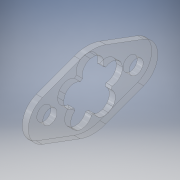
# Autodesk Inventor part: Ball Bearing Center
Saved by Autodesk Inventor 2017 (Build 210142000, 142)
## iProperties
Created: 2018-05-11
Part Number: Ball Bearing Center
Material: Polycarbonate, Clear
Document SubType Name: Modeling
Designer: Steven
Density: 1.2 g/cm^3
Appearance: Polycarbonate - Clear
Author: Steven
Autodesk Inventor part; units mm, degrees
ref_plane "YZ Plane" through (0, 0, 0) normal (1, 0, 0) x (0, 1, 0)
ref_plane "XZ Plane" through (0, 0, 0) normal (0, 1, 0) x (-1, 0, 0)
ref_plane "XY Plane" through (0, 0, 0) normal (0, 0, 1) x (1, 0, 0)
sketch "Sketch1" plane through (0, 0, 0) normal (1, 0, 0) x (0, 1, 0)
  circle A0 centre (0, 0) radius 8.89
  circle A1 centre (0, 0) radius 10.795 construction
  line L0 (0, 0) -> (0, 12.7)
  line L1 (0, 0) -> (0, -12.7)
  circle A2 centre (0, -12.7) radius 2.0955
  circle A3 centre (0, 12.7) radius 2.0955
  circle A4 centre (0, 12.7) radius 6.35 construction
  circle A5 centre (0, -12.7) radius 6.35 construction
  line L2 (5.9484, 14.9225) -> (10.1122, 3.7782)
  line L3 (10.1122, -3.7783) -> (5.9484, -14.9225)
  line L4 (-5.9484, -14.9225) -> (-10.1122, -3.7782)
  line L5 (-5.9484, 14.9225) -> (-10.1122, 3.7782)
  arc A6 (5.9484, 14.9225) -> (-5.9484, 14.9225) centre (0, 12.7) ccw
  arc A7 (10.1122, -3.7783) -> (10.1122, 3.7782) centre (0, 0) ccw
  arc A8 (-5.9484, -14.9225) -> (5.9484, -14.9225) centre (0, -12.7) ccw
  arc A9 (-10.1122, 3.7782) -> (-10.1122, -3.7782) centre (0, 0) ccw
  dimension "d0" = 17.78
  dimension "d1" = 21.59
  dimension "d2" = 12.7
  dimension "d3" = 12.7
  dimension "d4" = 4.191
  dimension "d5" = 4.191
  dimension "d6" = 12.7
  dimension "d7" = 12.7
  constraints: 16 point on circle, 14 tangent, 12 end point, 10 centre point, 6 coincident, 2 concentric, 2 vertical
  measures "d0" diameter of A0
  measures "d1" diameter of A1
  measures "d2" distance of L0.start L0.end
  measures "d3" distance of L0.start L1.end
  measures "d4" diameter of A2
  measures "d5" diameter of A3
  measures "d6" diameter of A4
  measures "d7" diameter of A5
extrude "Extrusion1" add sketch "Sketch1" along normal blind 1.778
sketch "Sketch2" plane through (1.778, 0, 0) normal (1, 0, 0) x (0, 0, -1)
  circle A0 centre (0, 0) radius 5.7785
  circle A1 centre (0, 5.7785) radius 3.175 construction
  circle A2 centre (-5.4957, 1.7857) radius 3.175 construction
  circle A3 centre (-3.3965, -4.6749) radius 3.175 construction
  circle A4 centre (3.3965, -4.6749) radius 3.175 construction
  circle A5 centre (5.4957, 1.7857) radius 3.175 construction
  circle A6 centre (0, 0) radius 8.89 projected
  arc A7 (-0.7829, 8.8555) -> (-8.1801, 3.4811) centre (0, 0) ccw
  arc A8 (8.1801, 3.4811) -> (0.7829, 8.8555) centre (0, 0) ccw
  arc A9 (5.8385, -6.704) -> (8.664, 1.9919) centre (0, 0) ccw
  arc A10 (-4.5717, -7.6244) -> (4.5717, -7.6244) centre (0, 0) ccw
  arc A11 (-8.664, 1.9919) -> (-5.8385, -6.704) centre (0, 0) ccw
  arc A12 (-8.664, 1.9919) -> (-5.6095, -1.3873) centre (-5.4957, 1.7857) ccw
  arc A13 (-5.3536, -2.1748) -> (-5.8385, -6.704) centre (-3.3965, -4.6749) ccw
  arc A14 (-4.5717, -7.6244) -> (-0.414, -5.7636) centre (-3.3965, -4.6749) ccw
  arc A15 (0.414, -5.7636) -> (4.5717, -7.6244) centre (3.3965, -4.6749) ccw
  arc A16 (5.8385, -6.704) -> (5.3536, -2.1748) centre (3.3965, -4.6749) ccw
  arc A17 (5.6095, -1.3873) -> (8.664, 1.9919) centre (5.4957, 1.7857) ccw
  arc A18 (8.1801, 3.4811) -> (3.7227, 4.4195) centre (5.4957, 1.7857) ccw
  arc A19 (3.0528, 4.9062) -> (0.7829, 8.8555) centre (0, 5.7785) ccw
  arc A20 (-0.7829, 8.8555) -> (-3.0528, 4.9062) centre (0, 5.7785) ccw
  arc A21 (-3.7227, 4.4195) -> (-8.1801, 3.4811) centre (-5.4957, 1.7857) ccw
  dimension "d10" = 11.557
  dimension "d11" = 6.35
  dimension "d14" = 360
  constraints: 50 point on circle, 20 centre point, 5 concentric, 1 coincident, 35 other
  measures "d11" diameter of A1
extrude "Extrusion2" add sketch "Sketch2" against normal blind 1.778 contours A0 A19 A6 A18 | A17 A6 A16 A0 | A0 A21 A6 A20 | A15 A6 A14 A0 | A0 A13 A6 A12
body "Solid1"
